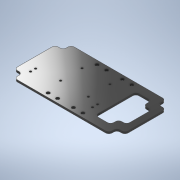
# Autodesk Inventor part: Sole_frame
Saved by Autodesk Inventor 2022.3 (Build 263350000, 350)
## iProperties
Part Number: Sole_frame
Material: GFRP
Document SubType Name: Modeling
Designer: Masato Kubotera
Density: 1.75 g/cm^3
Appearance: 低 光沢 - 黒
Description: GFRP T3
Mass: 59.3319 g
Surface Area: 254.466 cm^2
Volume: 33.904 cm^3
Author: Masato Kubotera
Autodesk Inventor part; units mm, degrees
ref_plane "YZ Plane" through (0, 0, 0) normal (1, 0, 0) x (0, 1, 0)
ref_plane "XZ Plane" through (0, 0, 0) normal (0, 1, 0) x (-1, 0, 0)
ref_plane "XY Plane" through (0, 0, 0) normal (0, 0, 1) x (1, 0, 0)
sketch "スケッチ1" plane through (0, 0, 0) normal (0, 0, 1) x (1, 0, 0)
  line L0 (-96.735, 64.25) -> (78.265, 64.25)
  line L1 (78.265, 64.25) -> (78.265, -25.75)
  line L2 (78.265, -25.75) -> (-96.735, -25.75)
  line L3 (-96.735, -25.75) -> (-96.735, 64.25)
  line L4 (-96.735, 64.25) -> (78.265, -25.75) construction
  line L5 (78.265, 64.25) -> (-96.735, -25.75) construction
  line L6 (-96.735, 19.25) -> (78.265, 19.25) construction
  line L7 (-96.735, 0) -> (78.265, 0) construction
  line L8 (-80, 4) -> (-80, -4) construction
  circle A0 centre (-80, -4) radius 1.6
  line L9 (0, 64.25) -> (0, -25.75) construction
  line L10 (18, -4) -> (18, 4) construction
  circle A1 centre (18, -4) radius 1.6
  circle A2 centre (-80, 4) radius 1.6
  circle A3 centre (18, 4) radius 1.6
  line L11 (15, 12.5) -> (21, 12.5) construction
  line L12 (21, 12.5) -> (21, -12.5) construction
  line L13 (21, -12.5) -> (15, -12.5) construction
  line L14 (15, -12.5) -> (15, 12.5) construction
  line L15 (15, 12.5) -> (21, -12.5) construction
  line L16 (21, 12.5) -> (15, -12.5) construction
  line L17 (-83, 12.5) -> (-77, 12.5) construction
  line L18 (-77, 12.5) -> (-77, -12.5) construction
  line L19 (-77, -12.5) -> (-83, -12.5) construction
  line L20 (-83, -12.5) -> (-83, 12.5) construction
  line L21 (-83, 12.5) -> (-77, -12.5) construction
  line L22 (-77, 12.5) -> (-83, -12.5) construction
  line L23 (-67, 49.25) -> (5, 49.25) construction
  line L24 (5, 49.25) -> (5, -10.75) construction
  line L25 (5, -10.75) -> (-67, -10.75) construction
  line L26 (-67, -10.75) -> (-67, 49.25) construction
  line L27 (-67, 49.25) -> (5, -10.75) construction
  line L28 (5, 49.25) -> (-67, -10.75) construction
  line L29 (-83, -4.5) -> (-83, 20.5) construction
  line L30 (-83, 20.5) -> (-77, 20.5) construction
  line L31 (-77, 20.5) -> (-77, -4.5) construction
  line L32 (-77, -4.5) -> (-83, -4.5) construction
  circle A4 centre (-80, 12) radius 1.6
  circle A5 centre (-80, 4) radius 1.6
  line L33 (15, 20.5) -> (21, 20.5) construction
  line L34 (15, -4.5) -> (15, 20.5) construction
  line L35 (21, -4.5) -> (15, -4.5) construction
  line L36 (21, 20.5) -> (21, -4.5) construction
  circle A6 centre (18, 4) radius 1.6
  circle A7 centre (18, 12) radius 1.6
  line L37 (-83, 3.5) -> (-83, 28.5) construction
  line L38 (-83, 28.5) -> (-77, 28.5) construction
  line L39 (-77, 28.5) -> (-77, 3.5) construction
  line L40 (-77, 3.5) -> (-83, 3.5) construction
  circle A8 centre (-80, 20) radius 1.6
  circle A9 centre (-80, 12) radius 1.6
  line L41 (15, 28.5) -> (21, 28.5) construction
  line L42 (15, 3.5) -> (15, 28.5) construction
  line L43 (21, 3.5) -> (15, 3.5) construction
  line L44 (21, 28.5) -> (21, 3.5) construction
  circle A10 centre (18, 12) radius 1.6
  circle A11 centre (18, 20) radius 1.6
  circle A12 centre (-80, -12) radius 1.6
  line L45 (-77, -20.5) -> (-83, -20.5) construction
  line L46 (-83, -20.5) -> (-83, 4.5) construction
  line L47 (-77, 4.5) -> (-77, -20.5) construction
  line L48 (15, -20.5) -> (15, 4.5) construction
  circle A13 centre (18, -12) radius 1.6
  line L49 (21, -20.5) -> (15, -20.5) construction
  line L50 (21, 4.5) -> (21, -20.5) construction
  line L51 (-1.735, -25.75) -> (78.265, -25.75) construction
  line L52 (78.265, -25.75) -> (78.265, -13.05) construction
  line L53 (78.265, -13.05) -> (-1.735, -13.05) construction
  line L54 (-1.735, -13.05) -> (-1.735, -25.75) construction
  line L55 (-1.735, -25.75) -> (78.265, -13.05) construction
  line L56 (78.265, -25.75) -> (-1.735, -13.05) construction
  line L57 (78.265, -19.4) -> (-1.735, -19.4) construction
  line L58 (38.265, -25.75) -> (38.265, -13.05) construction
  circle A14 centre (3.265, -19.4) radius 2.6
  circle A15 centre (18.265, -19.4) radius 2.6
  line L59 (76.765, -17.3793) -> (76.765, -21.4207) construction
  line L60 (76.765, -21.4207) -> (73.265, -23.4415) construction
  line L61 (73.265, -23.4415) -> (69.765, -21.4207) construction
  line L62 (69.765, -21.4207) -> (69.765, -17.3793) construction
  line L63 (69.765, -17.3793) -> (73.265, -15.3585) construction
  line L64 (73.265, -15.3585) -> (76.765, -17.3793) construction
  line L65 (-9.235, 64.25) -> (-9.235, -25.75) construction
  circle A16 centre (3.265, 57.9) radius 2.6
  circle A17 centre (18.265, 57.9) radius 2.6
  line L66 (76.765, 55.8793) -> (76.765, 59.9207) construction
  line L67 (76.765, 59.9207) -> (73.265, 61.9415) construction
  line L68 (73.265, 61.9415) -> (69.765, 59.9207) construction
  line L69 (69.765, 59.9207) -> (69.765, 55.8793) construction
  line L70 (69.765, 55.8793) -> (73.265, 53.8585) construction
  line L71 (73.265, 53.8585) -> (76.765, 55.8793) construction
  circle A18 centre (-21.735, -19.4) radius 2.6
  circle A19 centre (-36.735, -19.4) radius 2.6
  line L72 (-95.235, -17.3793) -> (-95.235, -21.4207) construction
  line L73 (-95.235, -21.4207) -> (-91.735, -23.4415) construction
  line L74 (-91.735, -23.4415) -> (-88.235, -21.4207) construction
  line L75 (-88.235, -21.4207) -> (-88.235, -17.3793) construction
  line L76 (-88.235, -17.3793) -> (-91.735, -15.3585) construction
  line L77 (-91.735, -15.3585) -> (-95.235, -17.3793) construction
  circle A20 centre (-21.735, 57.9) radius 2.6
  circle A21 centre (-36.735, 57.9) radius 2.6
  line L78 (-88.235, 55.8793) -> (-91.735, 53.8585) construction
  line L79 (-88.235, 59.9207) -> (-88.235, 55.8793) construction
  line L80 (-91.735, 61.9415) -> (-88.235, 59.9207) construction
  line L81 (-95.235, 59.9207) -> (-91.735, 61.9415) construction
  line L82 (-95.235, 55.8793) -> (-95.235, 59.9207) construction
  line L83 (-91.735, 53.8585) -> (-95.235, 55.8793) construction
  line L84 (-46.735, 44.25) -> (3.265, 44.25)
  line L85 (3.265, 44.25) -> (3.265, 4.25)
  line L86 (3.265, 4.25) -> (-46.735, 4.25)
  line L87 (-46.735, 4.25) -> (-46.735, 44.25)
  line L88 (-46.735, 44.25) -> (3.265, 4.25) construction
  line L89 (3.265, 44.25) -> (-46.735, 4.25) construction
  line L90 (-43.735, 41.25) -> (0.265, 41.25) construction
  line L91 (0.265, 41.25) -> (0.265, 7.25) construction
  line L92 (0.265, 7.25) -> (-43.735, 7.25) construction
  line L93 (-43.735, 7.25) -> (-43.735, 41.25) construction
  line L94 (-43.735, 41.25) -> (0.265, 7.25) construction
  line L95 (0.265, 41.25) -> (-43.735, 7.25) construction
  circle A22 centre (-43.735, 7.25) radius 1.6
  circle A23 centre (-43.735, 41.25) radius 1.6
  circle A24 centre (0.265, 41.25) radius 1.6
  circle A25 centre (0.265, 7.25) radius 1.6
  line L96 (78.265, -13.05) -> (65.565, -13.05)
  line L97 (65.565, -13.05) -> (65.565, -25.75)
  line L98 (78.265, 51.55) -> (65.565, 51.55)
  line L99 (65.565, 51.55) -> (65.565, 64.25)
  line L100 (-96.735, -13.05) -> (-84.035, -13.05)
  line L101 (-84.035, -13.05) -> (-84.035, -25.75)
  line L102 (-84.035, 51.55) -> (-84.035, 64.25)
  line L103 (-96.735, 51.55) -> (-84.035, 51.55)
  line L104 (-62, -13.05) -> (-61.735, -13.05)
  line L105 (-56.735, -8.05) -> (-56.735, 46.55)
  line L106 (-61.735, 51.55) -> (-62, 51.55)
  line L107 (-67, 46.55) -> (-67, -8.05)
  line L108 (-67, -13.05) -> (-56.735, 51.55) construction
  line L109 (-56.735, -13.05) -> (-67, 51.55) construction
  arc A26 (-67, -8.05) -> (-62, -13.05) centre (-62, -8.05) ccw
  arc A27 (-61.735, -13.05) -> (-56.735, -8.05) centre (-61.735, -8.05) ccw
  arc A28 (-56.735, 46.55) -> (-61.735, 51.55) centre (-61.735, 46.55) ccw
  arc A29 (-62, 51.55) -> (-67, 46.55) centre (-62, 46.55) ccw
  line L110 (50.565, 51.55) -> (36, 51.55)
  line L111 (31, 46.55) -> (31, -8.05)
  line L112 (36, -13.05) -> (50.565, -13.05)
  line L113 (55.565, -8.05) -> (55.565, -5.35)
  line L114 (55.565, 51.55) -> (31, -13.05) construction
  line L115 (31, 51.55) -> (55.565, -13.05) construction
  line L116 (60.565, -0.35) -> (63.265, -0.35)
  line L117 (68.265, 4.65) -> (68.265, 33.85)
  line L118 (63.265, 38.85) -> (60.565, 38.85)
  line L119 (55.565, 43.85) -> (55.565, 46.55)
  arc A30 (36, 51.55) -> (31, 46.55) centre (36, 46.55) ccw
  arc A31 (55.565, 46.55) -> (50.565, 51.55) centre (50.565, 46.55) ccw
  arc A32 (55.565, 43.85) -> (60.565, 38.85) centre (60.565, 43.85) ccw
  arc A33 (68.265, 33.85) -> (63.265, 38.85) centre (63.265, 33.85) ccw
  arc A34 (63.265, -0.35) -> (68.265, 4.65) centre (63.265, 4.65) ccw
  arc A35 (60.565, -0.35) -> (55.565, -5.35) centre (60.565, -5.35) ccw
  arc A36 (50.565, -13.05) -> (55.565, -8.05) centre (50.565, -8.05) ccw
  arc A37 (31, -8.05) -> (36, -13.05) centre (36, -8.05) ccw
  point P0 (0, 0)
  point P1 (-9.235, 19.25)
  point P2 (-80, 0)
  point P3 (18, 0)
  point P4 (-31, 19.25)
  point P5 (38.265, -19.4)
  point P6 (73.265, -19.4)
  point P7 (-21.735, 24.25)
  point P8 (-21.735, 24.25)
  point P9 (-21.735, 24.25)
  point P10 (-61.8675, 19.25)
  point P11 (43.2825, 19.25)
  point P12 (55.565, -0.35)
  point P13 (55.565, 38.85)
  point P14 (68.265, 19.25)
  dimension "d0" = 175
  dimension "d1" = 90
  dimension "d2" = 25.75
  dimension "d3" = 3.2
  dimension "d4" = 8
  dimension "d5" = 8
  dimension "d6" = 3.2
  dimension "d16" = 78.265
  dimension "d17" = 6
  dimension "d18" = 25
  dimension "d19" = 21
  dimension "d20" = 6
  dimension "d21" = 25
  dimension "d22" = 104
  dimension "d23" = 15
  dimension "d24" = 15
  dimension "d25" = 10
  dimension "d26" = 10
  dimension "d57" = 8
  dimension "d64" = 8
  dimension "d69" = 80
  dimension "d70" = 12.7
  dimension "d71" = 5.2
  dimension "d72" = 5.2
  dimension "d73" = 15
  dimension "d74" = 20
  dimension "d75" = 7
  dimension "d76" = 35
  dimension "d77" = 0
  dimension "d78" = 0
  dimension "d79" = 50
  dimension "d80" = 40
  dimension "d81" = 44
  dimension "d82" = 34
  dimension "d83" = 3.2
  dimension "d84" = 3.2
  dimension "d85" = 3.2
  dimension "d86" = 3.2
  dimension "d87" = 12.7
  dimension "d88" = 5
  dimension "d89" = 100
  dimension "d91" = 64.6
  dimension "d92" = 12.7
  dimension "d93" = 10
  dimension "d94" = 10
  dimension "d95" = 10.265
  dimension "d96" = 5
  dimension "d97" = 10
  dimension "d98" = 10
  dimension "d99" = 12.7
  dimension "d100" = 10
  dimension "d101" = 5
  constraints: 240 end point, 38 centre point, 38 point on line, 35 symmetric about line, 31 midpoint, 24 point on circle, 24 tangent, 21 parallel, 14 perpendicular, 10 equal radius, 10 horizontal, 6 coincident, 4 vertical, 3 collinear, 85 other
  measures "d0" distance of L1.end L2.end
  measures "d1" distance of L0.end L1.end
  measures "d2" distance of L2.end L7.start
  measures "d3" diameter of A0
  measures "d4" distance of L8.start L8.end
  measures "d5" distance of L10.start L10.end
  measures "d6" diameter of A1
  measures "d16" distance of L0.end L9.start
  measures "d17" distance of L12.end L13.end
  measures "d18" distance of L11.end L12.end
  measures "d19" horizontal distance of L11.end point (0, 0)
  measures "d20" distance of L18.end L19.end
  measures "d21" distance of L17.end L18.end
  measures "d22" distance of L12.end L19.end
  measures "d23" distance between parallel lines of L23 L0
  measures "d24" distance between parallel lines of L2 L25
  measures "d25" distance between parallel lines of L26 L18
  measures "d26" distance between parallel lines of L14 L24
  measures "d57" distance of L19.end L29.start
  measures "d64" distance of A0.centre A12.centre
  measures "d69" distance of L51.start L51.end
  measures "d70" distance of L53.end L51.start
  measures "d71" diameter of A14
  measures "d72" diameter of A15
  measures "d73" distance of A15.centre A14.centre
  measures "d74" distance from line of L58 A15.centre
  measures "d75" distance between parallel lines of L61 L64
  measures "d76" distance from line of point (73.265, -19.4) L58
  measures "d77" distance between parallel lines of L51 L2
  measures "d78" distance between parallel lines of L1 L52
  measures "d79" distance of L85.end L86.end
  measures "d80" distance of L84.end L85.end
  measures "d81" distance of L91.end L92.end
  measures "d82" distance of L90.end L91.end
  measures "d83" diameter of A22
  measures "d84" diameter of A23
  measures "d85" diameter of A24
  measures "d86" diameter of A25
  measures "d87" distance of L97.end L1.end
  measures "d88" distance from line of L6 point (-21.735, 24.25)
  measures "d89" distance from line of point (-21.735, 24.25) L1
  measures "d91" distance of L109.end L108.start
  measures "d92" distance between parallel lines of L0 L106
  measures "d93" distance between parallel lines of L107 L39
  measures "d94" distance between parallel lines of L87 L105
  measures "d95" distance of L108.start L109.start
  measures "d96" radius of A26
  measures "d97" distance between parallel lines of L44 L111
  measures "d98" distance between parallel lines of L113 L97
  measures "d99" distance between parallel lines of L116 L96
  measures "d100" distance between parallel lines of L117 L1
  measures "d101" radius of A30
extrude "押し出し1" add sketch "スケッチ1" along normal blind 3 contours L0 L99 L98 L1 L96 L97 L2 L101 L100 L3 L103 L102 | A4 | A7 | A8 | A11 | A12 | A13 | L84 L85 L86 L87 | A26 L107 A29 L106 A28 L105 A27 L104
fillet "フィレット1" radius 5 12 edges at (65.565, 64.25, 1.5) (65.565, 51.55, 1.5) (78.265, 51.55, 1.5) (65.565, -13.05, 1.5) (78.265, -13.05, 1.5) (65.565, -25.75, 1.5) (-96.735, -13.05, 1.5) (-84.035, -13.05, 1.5) (-84.035, -25.75, 1.5) (-84.035, 64.25, 1.5) (-84.035, 51.55, 1.5) (-96.735, 51.55, 1.5)
equation "\"d3\" = d6"
equation "\"d4\" = d5"
equation "\"d20\" = d17"
equation "\"d21\" = d18"
